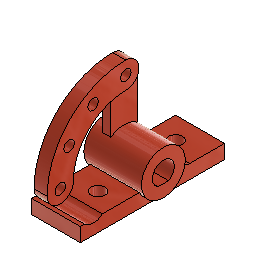
Design 11 v1 (Autodesk Fusion 360 design; units mm, degrees)
Autodesk Fusion 360 part; units mm, degrees
note: some values were not read from the file. Set by a fixed rule: which sketch regions a step uses.
sketch "Sketch1" plane through (0, 0, 0) normal (1, 0, 0) x (0, 1, 0)
  line L0 (825, -80) -> (-825, -80)
  line L1 (-825, -80) -> (-825, 80)
  line L2 (-825, 80) -> (825, 80)
  line L3 (825, 80) -> (825, -80)
  line L4 (825, -80) -> (-825, 80) construction
  line L5 (-825, -80) -> (825, 80) construction
  circle A0 centre (75, 190) radius 125
  circle A1 centre (75, 190) radius 250
  arc A2 (75, 790) -> (-525, 190) centre (75, 190) ccw
  arc A3 (75, 1090) -> (-825, 190) centre (75, 190) ccw
  circle A4 centre (75, 940) radius 150
  circle A5 centre (-675, 190) radius 150
  circle A6 centre (75, 940) radius 60
  circle A7 centre (-300, 839.5191) radius 60
  circle A8 centre (-574.5191, 565) radius 60
  circle A9 centre (-675, 190) radius 60
  line L6 (225, 940) -> (225, 390)
  line L7 (-75, 940) -> (-75, 390)
  point P0 (-574.5191, -185)
  point P1 (724.5191, -185)
  dimension "d1" = 1650
  dimension "d2" = 160
  dimension "d3" = 250
  dimension "d4" = 500
  dimension "d5" = 270
  dimension "d6" = 75
  dimension "d7" = 600
  dimension "d8" = 900
  dimension "d9" = 120
  dimension "d11" = 360
  dimension "d13" = 90
  constraint horizontal L0
  constraint perpendicular L0 L1
  constraint parallel L0 L2
  constraint parallel L1 L3
  constraint coincident L4 origin
  constraint coincident L5 origin
  constraint concentric A0 A1
  constraint coincident A0.centre A1.centre
  constraint coincident A3.start A4
  constraint tangent A3 A4
  constraint coincident A2.start A4
  constraint coincident A3.end A5
  constraint tangent A3 A5
  constraint coincident A2.end A5
  constraint concentric A4 A6
  constraint coincident A4 L6.start
  constraint coincident A1 L6.end
  constraint tangent A4 L6
  constraint vertical L6
  constraint coincident A4 L7.start
  constraint coincident A1 L7.end
  constraint tangent A4 L7
  constraint vertical L7
  measures "d1" distance of L1.end L2.end
  measures "d2" distance of L0.end L1.end
  measures "d3" diameter of A0
  measures "d4" diameter of A1
  measures "d5" distance of L0 A0.centre
  measures "d6" horizontal distance of origin A0.centre
  measures "d7" radius of A2
  measures "d8" radius of A3
  measures "d9" diameter of A6
extrude "Extrude1" add sketch "Sketch1" along normal mid plane 560 contours L0 L1 L2 L3 A1 A5
extrude "Extrude2" add sketch "Sketch1" along normal mid plane 660 contours L2 A0 A1 | L2 A0 A1 | L2 A0 picked at (60.5747, 77.5767)
extrude "Extrude3" add sketch "Sketch1" against normal blind 150 from surface at -100 contours L2 A5 | L2 A5 | A2 A3 A4 A5 L7 | A4 | A2 A4 L7
extrude "Extrude4" add sketch "Sketch1" against normal blind 100 from surface at -120 contours A1 A2 A4 L6 L7
hole "Hole1" at (-30, 575, 80) direction (0, 0, -1) diameter 160 end through all
hole "Hole2" at (30, -373.0196, 80) direction (0, 0, -1) diameter 160 end through all
fillet "Fillet1" radius 100 1 edges at (0, 299.4994, 80)
